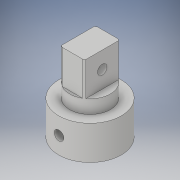
# Autodesk Inventor part: ДЗ2-1
Saved by Autodesk Inventor 2019 (Build 230136000, 136)
## iProperties
Created: 2020-04-16
Part Number: ДЗ2-1
Material: Типовые
Document SubType Name: Modeling
Designer: Ivan
Density: 1 g/cm^3
Appearance: По умолчанию
Mass: 57.7861 g
Surface Area: 112.559 cm^2
Volume: 57.7861 cm^3
Author: Ivan
Autodesk Inventor part; units mm, degrees
ref_plane "YZ Plane" through (0, 0, 0) normal (1, 0, 0) x (0, 1, 0)
ref_plane "XZ Plane" through (0, 0, 0) normal (0, 1, 0) x (-1, 0, 0)
ref_plane "XY Plane" through (0, 0, 0) normal (0, 0, 1) x (1, 0, 0)
sketch "Эскиз1" plane through (0, 0, 0) normal (0, 1, 0) x (-1, 0, 0)
  circle A0 centre (0, 0) radius 23
  dimension "d0" = 46
  constraints: 1 centre point, 1 coincident
  measures "d0" diameter of A0
extrude "Выдавливание1" add sketch "Эскиз1" along normal blind 25
sketch "Эскиз2" plane through (0, 25, 0) normal (0, 1, 0) x (1, 0, 0)
  circle A0 centre (0, 0) radius 15
  dimension "d3" = 30
  constraints: 1 centre point, 1 coincident
  measures "d3" diameter of A0
extrude "Выдавливание2" add sketch "Эскиз2" along normal blind 35
sketch "Эскиз3" plane through (0, 60, 0) normal (0, 1, 0) x (1, 0, 0)
  line L0 (9, -13) -> (-9, -13)
  line L1 (-9, -13) -> (-9, 13)
  line L2 (-9, 13) -> (9, 13)
  line L3 (9, 13) -> (9, -13)
  line L4 (9, -13) -> (-9, 13) construction
  line L5 (-9, -13) -> (9, 13) construction
  circle A0 centre (0, 0) radius 23 projected
  dimension "d6" = 26
  dimension "d7" = 18
  constraints: 12 end point, 2 midpoint, 2 parallel, 1 horizontal, 1 perpendicular
  measures "d6" distance between parallel lines of L2 L0
  measures "d7" distance between parallel lines of L3 L1
extrude "Выдавливание3" cut sketch "Эскиз3" against normal blind 25
sketch "Эскиз4" plane through (9, 60, 12) normal (1, 0, 0) x (0, 0, -1)
  circle A0 centre (12, -12.5) radius 3.5
  line L0 (0, -25) -> (24, -25) projected
  point P0 (12, -60)
  dimension "d10" = 7
  dimension "d11" = 12.5
  constraints: 1 centre point
  measures "d10" diameter of A0
  measures "d11" distance from line of L0 A0.centre
extrude "Выдавливание4" cut sketch "Эскиз4" along normal through all both and the other way through all
sketch "Эскиз5" plane through (0, 0, 0) normal (0, 0, 1) x (1, 0, 0)
  circle A0 centre (0, 12.5) radius 3.5
  point P0 (0, 0)
  dimension "d14" = 7
  dimension "d15" = 12.5
  constraints: 1 centre point
  measures "d14" diameter of A0
  measures "d15" distance of point (0, 0) A0.centre
extrude "Выдавливание5" cut sketch "Эскиз5" along normal through all both and the other way through all
